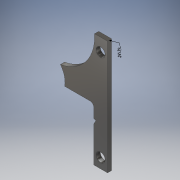
# Autodesk Inventor part: 1-4inch_FixedKnifeBig_Piece1
Saved by Autodesk Inventor 2018 (Build 220112000, 112)
## iProperties
Created: 2018-01-21
Part Number: 1-4inch_FixedKnifeBig_Piece1
Material: Generic
Document SubType Name: Modeling
Designer: Olivier
Density: 1 g/cm^3
Appearance: Default
Author: Olivier
Autodesk Inventor part; units mm, degrees
ref_plane "YZ Plane" through (0, 0, 0) normal (1, 0, 0) x (0, 1, 0)
ref_plane "XZ Plane" through (0, 0, 0) normal (0, 1, 0) x (-1, 0, 0)
ref_plane "XY Plane" through (0, 0, 0) normal (0, 0, 1) x (1, 0, 0)
sketch "Sketch1" plane through (0, 0, 0) normal (0, 0, 1) x (1, 0, 0)
  arc A0 (-54.4767, 14.3972) -> (-15, 60) centre (-62.8769, 61.5571) ccw
  arc A1 (-49.5719, -5) -> (-54.4767, 14.3972) centre (-74.5236, -0.9906) ccw
  line L0 (-49.5719, -5) -> (-20, -5)
  arc A2 (-16, -9) -> (-20, -5) centre (-20, -9) ccw
  line L1 (-16, -9) -> (-16, -20.3999)
  line L2 (-16, -20.3999) -> (-13.5, -21.5)
  line L3 (-13.5, -21.5) -> (-16, -25.9706)
  line L4 (-16, -25.9706) -> (-16, -67)
  line L5 (-16, -67) -> (0, -67)
  line L6 (0, -67) -> (0, 65)
  line L7 (0, 65) -> (-15, 65)
  line L8 (-15, 65) -> (-15, 60)
  circle A3 centre (-8, 50) radius 5.25
  circle A4 centre (-8, -55.4085) radius 5.25
  arc A5 (-54.4767, 14.3972) -> (-15, 60) centre (-62.8769, 61.5571) ccw
  arc A6 (-49.5719, -5) -> (-54.4767, 14.3972) centre (-74.5236, -0.9906) ccw
  line L9 (-49.5719, -5) -> (-20, -5)
  arc A7 (-16, -9) -> (-20, -5) centre (-20, -9) ccw
  line L10 (-16, -9) -> (-16, -20.3999)
  line L11 (-16, -20.3999) -> (-13.5, -21.5)
  line L12 (-13.5, -21.5) -> (-16, -25.9706)
  line L13 (-16, -25.9706) -> (-16, -67)
  line L14 (-16, -67) -> (0, -67)
  line L15 (0, -67) -> (0, 65)
  line L16 (0, 65) -> (-15, 65)
  line L17 (-15, 65) -> (-15, 60)
  circle A8 centre (-8, 50) radius 5.25
  circle A9 centre (-8, -55.4085) radius 5.25
  point P0 (0, 0)
  constraints: 36 end point, 12 point on circle, 10 centre point
extrude "Extrusion1" add sketch "Sketch1" along normal blind 4.7625
body "Solid1"
